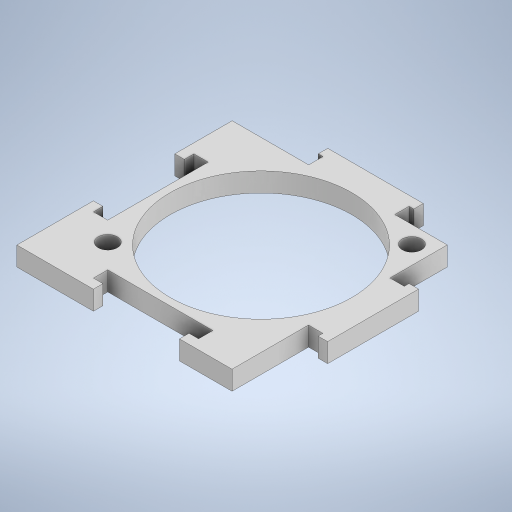
# Autodesk Inventor part: Maschio-femmina
Saved by Autodesk Inventor 2024 (Build 280153000, 153)
## iProperties
Created: 2024-01-14
Part Number: Maschio-femmina
Material: Generico
Document SubType Name: Modeling
Designer: Leonardo
Density: 1 g/cm^3
Appearance: Default
Author: Leonardo
Autodesk Inventor part; units mm, degrees
ref_plane "YZ Plane" through (0, 0, 0) normal (1, 0, 0) x (0, 1, 0)
ref_plane "XZ Plane" through (0, 0, 0) normal (0, 1, 0) x (-1, 0, 0)
ref_plane "XY Plane" through (0, 0, 0) normal (0, 0, 1) x (1, 0, 0)
sketch "Schizzo1" plane through (0, 0, 0) normal (0, 1, 0) x (-1, 0, 0)
  line L0 (10.0009, -10.0148) -> (9.0009, -10.0148)
  line L1 (-10, 9) -> (-10, 10)
  line L2 (-10, 12) -> (-10, 10)
  line L3 (-10, -10.0148) -> (-9, -10.0148)
  line L4 (9.0009, -10.0148) -> (8.0009, -10.0148)
  line L5 (-9, -10.0148) -> (-8, -10.0148)
  line L6 (-10, 9) -> (-10, 8)
  line L7 (-10, -10.0148) -> (-10, -7.7324)
  circle A0 centre (-0.2724, -0.2591) radius 9.5
  line L8 (12.5009, -8.0148) -> (12.5009, -10.0148)
  line L9 (12.5009, -10.0148) -> (10.0009, -10.0148)
  line L10 (12.5009, 7.9852) -> (12.5009, 9.9852)
  line L11 (8, 12.5) -> (10, 12.5)
  line L12 (12.5009, 9.9852) -> (12.5009, 12.5)
  line L13 (12.5009, 12.5) -> (10, 12.5)
  line L14 (-8, 12.5) -> (-10, 12.5)
  line L15 (-10, 12.5) -> (-10, 12)
  line L16 (8.0009, -10.0148) -> (7.5009, -10.0148)
  line L17 (-8, -10.0148) -> (-7.5, -10.0148)
  circle A1 centre (-8.1016, -8.2148) radius 1
  circle A2 centre (8.0009, 7.5) radius 1
  line L18 (12.5009, -7.0148) -> (12.5009, -8.0148)
  line L19 (-7, 12.5) -> (-8, 12.5)
  line L20 (7.5009, -10.0148) -> (4.5009, -10.0148)
  line L21 (-7.5, -10.0148) -> (-4.5, -10.0148)
  line L22 (4.5009, -11.5148) -> (5.0009, -11.5148)
  line L23 (5.0009, -11.5148) -> (5.0009, -12.5148)
  line L24 (4.5009, -11.5148) -> (4.5009, -10.0148)
  line L25 (-4.5, -11.5148) -> (-5, -11.5148)
  line L26 (-5, -11.5148) -> (-5, -12.5148)
  line L27 (-5, -12.5148) -> (5.0009, -12.5148)
  line L28 (-4.5, -11.5148) -> (-4.5, -10.0148)
  line L29 (4.5009, 11.5) -> (5.0009, 11.5)
  line L30 (-4.5, 12.5) -> (-7, 12.5)
  line L31 (5.0009, 10) -> (-4.5, 10)
  line L32 (-4.5, 11.5) -> (-5.5, 11.5)
  line L33 (-5.5, 11.5) -> (-5.5, 10)
  line L34 (-5.5, 10) -> (-4.5, 10)
  line L35 (-4.5, 11.5) -> (-4.5, 12.5)
  line L36 (4.5009, 11.5) -> (4.5009, 12.5)
  line L37 (4.5009, 11.5) -> (5.5009, 11.5)
  line L38 (5.5009, 11.5) -> (5.5009, 10)
  line L39 (5.5009, 10) -> (5.0009, 10)
  line L40 (8, 12.5) -> (4.5009, 12.5)
  line L41 (-10, -10.0148) -> (-10, -4.0148)
  line L42 (-10, 7.5) -> (-10, 4.5)
  line L43 (-10, 4.5) -> (-11.5, 4.5)
  line L44 (-11.5, 4.5) -> (-11.5, 5)
  line L45 (-11.5, 5) -> (-12.5, 5)
  line L46 (-10, -4.0148) -> (-11.5, -4.0148)
  line L47 (-11.5, -4.0148) -> (-11.5, -4.5148)
  line L48 (-11.5, -4.5148) -> (-12.5, -4.5148)
  line L49 (-10, 7.5) -> (-10, 8)
  line L50 (-12.5, 5) -> (-12.5, -4.5148)
  line L51 (12.5009, 4.5) -> (11.5009, 4.5)
  line L52 (11.5009, 4.5) -> (11.5009, 5.5)
  line L53 (11.5009, 5.5) -> (10.0009, 5.5)
  line L54 (12.5009, 4.5) -> (12.5009, 7.9852)
  line L55 (12.5009, -4.0148) -> (11.5009, -4.0148)
  line L56 (12.5009, -4.0148) -> (12.5009, -7.0148)
  line L57 (11.5009, -4.0148) -> (11.5009, -5.0148)
  line L58 (11.5009, -5.0148) -> (10.0009, -5.0148)
  line L59 (10.0009, -5.0148) -> (10.0009, 5.5)
  point P0 (0, 0)
  dimension "d45" = 2
  dimension "d54" = 2
  dimension "d56" = 0.5
  dimension "d59" = 0.5
  dimension "d72" = 2
  dimension "d81" = 3
  dimension "d82" = 0.5
  dimension "d83" = 0.5
  dimension "d87" = 1
  dimension "d90" = 0.5
  dimension "d92" = 0.5
  dimension "d93" = 1
  constraints: 120 end point, 14 perpendicular, 13 vertical, 10 horizontal, 3 centre point, 1 collinear, 1 point on line
  measures "d45" distance of L8.start L8.end
  measures "d54" distance of L14.start L14.end
  measures "d56" distance of L6.end L42.start
  measures "d59" distance of L5.end L17.end
  measures "d72" diameter of A1
  measures "d81" distance of L17.end L21.end
  measures "d82" distance of L22.start L22.end
  measures "d83" distance of L25.start L25.end
  measures "d87" distance of L29.start L37.end
  measures "d90" distance of L43.end L44.end
  measures "d92" distance of L46.end L47.end
  measures "d93" distance of L51.end L52.end
extrude "Estrusione6" add sketch "Schizzo1" along normal blind 2
